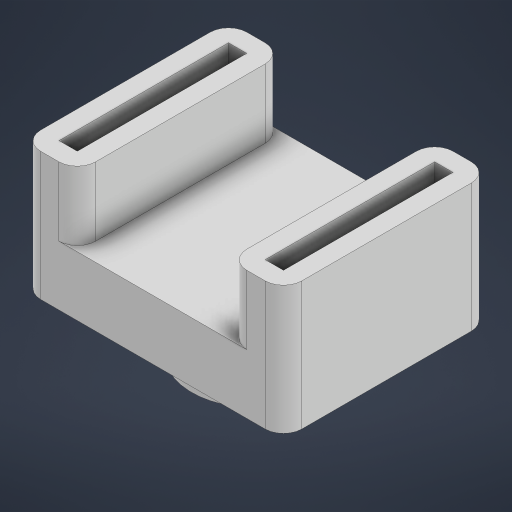
# Autodesk Inventor part: Keller
Saved by Autodesk Inventor 2023 (Build 270158030, 158C)
## iProperties
Created: 2022-05-18
Part Number: Keller
Material: Generic
Document SubType Name: Modeling
Designer: Simon
Density: 1 g/cm^3
Appearance: Default
Author: Simon
Autodesk Inventor part; units mm, degrees
ref_plane "YZ Plane" through (0, 0, 0) normal (1, 0, 0) x (0, 1, 0)
ref_plane "XZ Plane" through (0, 0, 0) normal (0, 1, 0) x (-1, 0, 0)
ref_plane "XY Plane" through (0, 0, 0) normal (0, 0, 1) x (1, 0, 0)
sketch "Sketch1" plane through (0, 0, 0) normal (0, 0, 1) x (1, 0, 0)
  line L0 (0, 0) -> (7, 0)
  line L1 (7, 0) -> (7, 7)
  line L2 (7, 7) -> (0, 7)
  line L3 (0, 7) -> (0, 0)
  line L4 (7, 0) -> (5.95, 0)
  line L5 (5.95, 0) -> (5.95, -4.3)
  line L6 (5.95, -4.3) -> (7, -4.3)
  line L7 (7, -4.3) -> (7, 0)
  dimension "d0" = 7
  dimension "d1" = 7
  dimension "d2" = 1.05
  dimension "d3" = 4.3
  constraints: 16 end point, 4 parallel, 2 horizontal, 2 perpendicular
  measures "d0" distance of L2.end L1.end
  measures "d1" distance of L1.end L0.end
  measures "d2" distance of L6.end L5.end
  measures "d3" distance of L5.end L4.end
revolve "Revolution1" add sketch "Sketch1" angle 360 about axis through (0, 7, 0) along (0, -1, 0)
sketch "Sketch2" plane through (0, 7, 0) normal (0, 1, 0) x (1, 0, 0)
  line L0 (-14.25, -11.25) -> (14.25, -11.25)
  line L1 (14.25, -11.25) -> (14.25, 11.25)
  line L2 (14.25, 11.25) -> (-14.25, 11.25)
  line L3 (-14.25, 11.25) -> (-14.25, -11.25)
  line L4 (-14.25, -11.25) -> (14.25, 11.25) construction
  line L5 (14.25, -11.25) -> (-14.25, 11.25) construction
  point P0 (0, 0)
  dimension "d5" = 28.5
  dimension "d6" = 22.5
  constraints: 12 end point, 2 midpoint, 2 parallel, 1 horizontal, 1 perpendicular
  measures "d5" distance of L2.end L1.end
  measures "d6" distance of L1.end L0.end
extrude "Extrusion1" add sketch "Sketch2" against normal blind 6.5
fillet "Fillet1" radius 2 4 edges at (-14.25, 3.75, 11.25) (-14.25, 3.75, -11.25) (14.25, 3.75, 11.25) (14.25, 3.75, -11.25)
sketch "Sketch3" plane through (-12.25, 7, -11.25) normal (0, 1, 0) x (1, 0, 0)
  arc A0 (26.5, -2) -> (24.5, 0) centre (24.5, -2) ccw projected
  line L0 (24.5, 0) -> (0, 0) projected
  arc A1 (0, 0) -> (-2, -2) centre (0, -2) ccw projected
  line L1 (-2, -2) -> (-2, -20.5) projected
  arc A2 (-2, -20.5) -> (0, -22.5) centre (0, -20.5) ccw projected
  line L2 (0, -22.5) -> (24.5, -22.5) projected
  arc A3 (24.5, -22.5) -> (26.5, -20.5) centre (24.5, -20.5) ccw projected
  line L3 (26.5, -20.5) -> (26.5, -2) projected
  line L4 (24.5, 0) -> (0, 0) projected
  line L5 (0, -22.5) -> (2, -22.5)
  line L6 (4, -20.5) -> (4, -2)
  line L7 (2, 0) -> (0, 0)
  line L8 (-2, -2) -> (-2, -20.5)
  arc A4 (0, 0) -> (-2, -2) centre (0, -2) ccw
  arc A5 (4, -2) -> (2, 0) centre (2, -2) ccw
  arc A6 (-2, -20.5) -> (0, -22.5) centre (0, -20.5) ccw
  arc A7 (2, -22.5) -> (4, -20.5) centre (2, -20.5) ccw
  line L9 (12.25, 1.2488) -> (12.25, 2.7237)
  arc A8 (26.5, -2) -> (24.5, 0) centre (24.5, -2) ccw
  line L10 (26.5, -2) -> (26.5, -20.5)
  arc A9 (24.5, -22.5) -> (26.5, -20.5) centre (24.5, -20.5) ccw
  line L11 (24.5, -22.5) -> (22.5, -22.5)
  line L12 (20.5, -20.5) -> (20.5, -2)
  line L13 (22.5, 0) -> (24.5, 0)
  line L14 (26.5, -2) -> (26.5, -20.5)
  arc A10 (26.5, -2) -> (24.5, 0) centre (24.5, -2) ccw
  arc A11 (22.5, 0) -> (20.5, -2) centre (22.5, -2) ccw
  arc A12 (24.5, -22.5) -> (26.5, -20.5) centre (24.5, -20.5) ccw
  arc A13 (20.5, -20.5) -> (22.5, -22.5) centre (22.5, -20.5) ccw
  line L15 (2, -2) -> (2, -20.5)
  line L16 (2, -20.5) -> (0, -20.5)
  line L17 (0, -20.5) -> (0, -2)
  line L18 (0, -2) -> (2, -2)
  line L19 (22.5, -2) -> (22.5, -20.5)
  line L20 (22.5, -20.5) -> (24.5, -20.5)
  line L21 (24.5, -20.5) -> (24.5, -2)
  line L22 (24.5, -2) -> (22.5, -2)
  point P0 (12.25, -11.25)
  point P1 (4, 0)
  point P2 (-2, 0)
  point P3 (20.5, 0)
  point P4 (26.5, 0)
  point P5 (2, 0)
  point P6 (2, -22.5)
  dimension "d10" = 6
  dimension "d11" = 2
  dimension "d12" = 2
  dimension "d13" = 2
  constraints: 36 end point, 20 point on circle, 20 symmetric about line, 10 centre point, 9 point on line, 8 tangent, 4 parallel, 3 equal radius, 2 perpendicular, 1 horizontal, 1 vertical, 12 other
  measures "d10" distance of point (-2, 0) point (4, 0)
  measures "d11" radius of A4
  measures "d12" distance between parallel lines of L6 L15
  measures "d13" distance between parallel lines of L12 L19
extrude "Extrusion2" add sketch "Sketch3" along normal blind 7.5 contours L3 A3 L2 A13 L12 A11 L0 A0 | A5 L6 A7 L2 A2 L1 A1 L0
body "Solid1"
